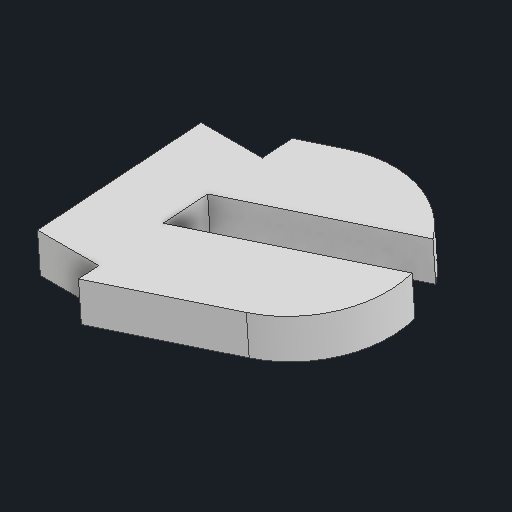
# Autodesk Inventor part: sponson_spanner_bottom_holder
Saved by Autodesk Inventor 2023 (Build 270158030, 158C)
## iProperties
Created: 2022-03-22
Part Number: sponson_spanner_bottom_holder
Material: Generic
Document SubType Name: Modeling
Designer: kardo
Density: 1 g/cm^3
Appearance: Default
Author: kardo
Autodesk Inventor part; units mm, degrees
ref_plane "YZ Plane" through (0, 0, 0) normal (1, 0, 0) x (0, 1, 0)
ref_plane "XZ Plane" through (0, 0, 0) normal (0, 1, 0) x (-1, 0, 0)
ref_plane "XY Plane" through (0, 0, 0) normal (0, 0, 1) x (1, 0, 0)
derived "parameters_frame.ipt"
derived "stencil_frame.ipt"
sketch "sk_joint_locations" plane through (81.12, 0, 0) normal (1, 0, 0) x (0, 1, 0)
  line L0 (0, 0) -> (111.39, 7.7891) construction
  line L1 (30.81, 28.832) -> (94.8, 28.832) construction
  arc A0 (30.81, 28.832) -> (9.48, 28.5282) centre (30.81, -720.1791) ccw construction
  line L2 (-254.1001, 21.0191) -> (9.48, 28.5282) construction
  line L3 (-363, 18.496) -> (-275.8801, 20.463) construction
  arc A1 (-275.8801, 20.463) -> (-254.1001, 21.0191) centre (-359.1231, 3707.4463) ccw construction
  line L4 (-210.8824, 4616.4994) -> (225.0382, -1617.4555) construction
  line L5 (-242.0001, 4592.9714) -> (-242.0001, -1605.7041) construction
  line L6 (-120.9999, 4592.9714) -> (-120.9999, -1605.7041) construction
  line L7 (-363, 4592.9714) -> (-363, -1605.7041) construction
  line L8 (0, 4592.9714) -> (0, -1605.7041) construction
  line L9 (551.8244, 47.4419) -> (-603.6686, 7.0912) construction
  line L10 (-657.8036, -26.1228) -> (709.4042, 69.4817) construction
  line L11 (178.2183, 30.3929) -> (177.9391, 38.388) construction
  line L12 (185.9231, 36.8959) -> (186.4825, 28.8959) construction
  line L13 (0, 6.528) -> (111.1168, 11.6964) construction
  line L14 (-242.0001, 45.8501) -> (-242.0001, 21.3638) construction
  line L15 (-363, 37.4293) -> (-363, 18.496) construction
  line L16 (-120.9999, 51.0063) -> (-120.9999, 24.811) construction
  line L17 (0, 52.89) -> (0, 28.2581) construction
  line L18 (108.3896, 50.6971) -> (108.935, 42.897) construction
  line L19 (109.4805, 35.0968) -> (108.935, 42.897) construction
  line L20 (109.4805, 35.0968) -> (110.0259, 27.2967) construction
  line L21 (110.0259, 27.2967) -> (110.5713, 19.4965) construction
  line L22 (110.5713, 19.4965) -> (111.1168, 11.6964) construction
  line L23 (0, 6.528) -> (0, 0) construction
  line L24 (94.8, 37.536) -> (94.8, 28.832) construction
  line L25 (94.8, 35.548) -> (94.8, 30.82) construction
  spline S0 degree 4 poles (-363, 37.4293) (-272.3626, 45.1427) (-181.5879, 49.7528) (-90.8131, 52.89) (0, 52.89) knots 0 0 0 0 0 1 1 1 1 1
  spline S1 degree 3 poles (0, 52.89) (86.3106, 52.89) (181.3207, 49.5034) (237, 36.448) knots 0 0 0 0 1 1 1 1
  spline S2 degree 2 poles (111.39, 7.7891) (176.0348, 12.3096) (237, 36.448) knots 0 0 0 1 1 1
  point P0 (-210.8824, 4616.4994)
  point P1 (225.0382, -1617.4555)
  point P2 (178.0787, 34.3904)
  point P3 (186.2028, 32.8959)
  point P4 (134.9575, 11.3411)
  point P5 (-363, 27.9627)
  point P6 (-242.0001, 33.6069)
  point P7 (-120.9999, 37.9086)
  point P8 (0, 40.5741)
  point P9 (94.8, 33.184)
derived "surface_body.ipt"
ref_plane "plane_tunnel_right" through (81.12, 0, 0) normal (1, 0, 0) x (0, 1, 0)
ref_plane "plane_sponson_boittom" through (126.048, 0, 0) normal (0.4037383, -0.0638184, 0.9126459) x (-0.1841621, 0.9714748, 0.1494022)
ref_plane "plane_base" through (81.12, 186.2028, 32.8959) normal (0, -0.9975641, -0.0697565) x (1, 0, 0)
sketch "sk_base" plane through (81.12, 186.2028, 32.8959) normal (0, -0.9975641, -0.0697565) x (1, 0, 0)
  line L0 (0, 4596.0046) -> (0, -1646.8096) projected
  line L1 (-1781.2929, 786.0927) -> (635.0064, -280.2312) construction
  line L2 (0, 4.0098) -> (3, 4.0098)
  line L3 (0, -4.0098) -> (3, -4.0098)
  line L4 (3, -4.0098) -> (3, -5.4715)
  line L5 (3, -5.4715) -> (4.8297, -6.279)
  line L6 (3, 4.0098) -> (3, 5.0098)
  line L7 (3, 5.0098) -> (8.7012, 2.4938)
  arc A0 (4.8297, -6.279) -> (8.7012, 2.4938) centre (6.7655, -1.8926) ccw
  line L8 (3, 0.8622) -> (11.4591, -2.8709)
  line L9 (8.7012, 2.4938) -> (4.8297, -6.279) construction
  line L10 (6.7655, -1.8926) -> (11.1519, -3.8283) construction
  line L11 (10.6517, -4.7006) -> (3, -1.3239)
  line L12 (3, 0.8622) -> (3, -1.3239)
  point P0 (-81.12, -19.8269)
  dimension "d3" = 3
  dimension "d4" = 2
  dimension "d5" = 1
  dimension "d6" = 2
  constraints: 22 end point, 6 parallel, 5 point on circle, 4 point on line, 2 perpendicular, 2 tangent, 1 centre point, 1 collinear, 1 other
  measures "d3" distance between parallel lines of L0 L6
  measures "d4" distance between parallel lines of L1 L8
  measures "d5" distance of L2.end L6.end
  measures "d6" distance of L4.end L5.end
extrude "thicken" add sketch "sk_base" along normal blind 2 contours L2 L6 L7 A0 L8 L12 L11 L5 L4 L3 L0
equation "\"d3\" = stringer_thickness"
equation "\"d4\" = bulkhead_thickness"
equation "\"d5\" = 0.5 * bulkhead_thickness"
equation "\"d6\" = bulkhead_thickness"
equation "\"d7\" = bulkhead_thickness"
equation "\"stringer_thickness\" = 3"
equation "\"bulkhead_thickness\" = 2"
body "Solid1"
